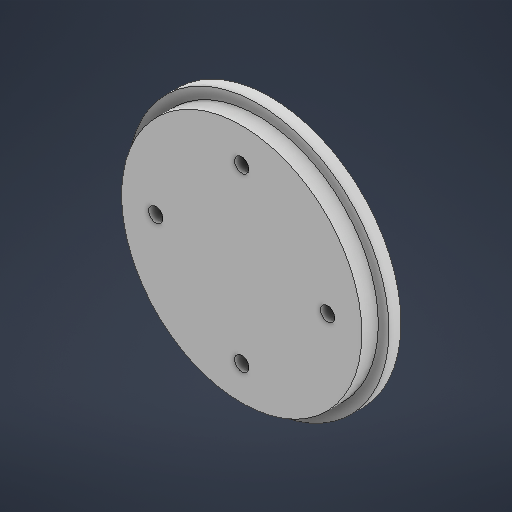
# Autodesk Inventor part: Fix_toDown_bearing
Saved by Autodesk Inventor 2025.2 (Build 292293000, 293)
## iProperties
Created: 2025-07-10
Part Number: Fix_toDown_bearing
Material: Generic
Document SubType Name: Modeling
Designer: Tiago
Density: 1 g/cm^3
Appearance: Default
Author: Tiago
Autodesk Inventor part; units mm, degrees
ref_plane "YZ Plane" through (0, 0, 0) normal (1, 0, 0) x (0, 1, 0)
ref_plane "XZ Plane" through (0, 0, 0) normal (0, 1, 0) x (-1, 0, 0)
ref_plane "XY Plane" through (0, 0, 0) normal (0, 0, 1) x (1, 0, 0)
sketch "Sketch1" plane through (0, 0, 0) normal (0, 0, 1) x (1, 0, 0)
  circle A0 centre (0, 0) radius 34.925
  circle A1 centre (0, 0) radius 38
  circle A2 centre (-25, 0) radius 2.1
  circle A3 centre (0, -25) radius 2.1
  circle A4 centre (25, 0) radius 2.1
  circle A5 centre (0, 25) radius 2.1
  dimension "d0" = 69.85
  dimension "d1" = 76
  dimension "d6" = 25
  dimension "d7" = 4.2
  dimension "d10" = 360
  constraints: 6 centre point, 2 coincident, 1 horizontal alignment, 9 other
  measures "d0" diameter of A0
  measures "d1" diameter of A1
  measures "d6" distance of point (0, 0) A2.centre
  measures "d7" diameter of A2
extrude "Extrusion1" add sketch "Sketch1" along normal blind 4.8 contours A0
extrude "Extrusion2" add sketch "Sketch1" against normal blind 3.5 contours A0 | A1
body "Solid1"
